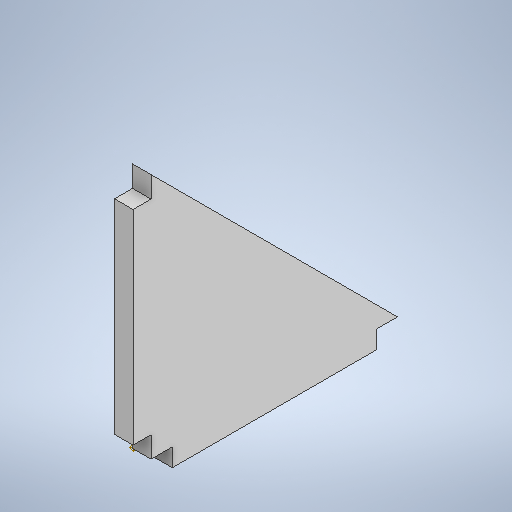
# Autodesk Inventor part: supporter
Saved by Autodesk Inventor 2025 (Build 290162000, 162)
## iProperties
Created: 2024-04-06
Part Number: supporter
Material: 일반
Document SubType Name: Modeling
Designer: gmsee
Density: 1 g/cm^3
Appearance: 기본값
Author: gmsee
Autodesk Inventor part; units mm, degrees
ref_plane "YZ Plane" through (0, 0, 0) normal (1, 0, 0) x (0, 1, 0)
ref_plane "XZ Plane" through (0, 0, 0) normal (0, 1, 0) x (-1, 0, 0)
ref_plane "XY Plane" through (0, 0, 0) normal (0, 0, 1) x (1, 0, 0)
sketch "스케치1" plane through (0, 0, 0) normal (1, 0, 0) x (0, 1, 0)
  line L0 (0, -46.5) -> (46.5, 0)
  line L1 (0, -4) -> (-3.4, -4)
  line L2 (-3.4, -4) -> (-3.4, -42.5)
  line L3 (-3.4, -42.5) -> (0, -42.5)
  line L4 (0, 0) -> (0, -4)
  line L5 (0, -42.5) -> (0, -46.5)
  line L6 (42.5, 0) -> (42.5, 3.4)
  line L7 (42.5, 3.4) -> (4, 3.4)
  line L8 (4, 3.4) -> (4, 0)
  line L9 (46.5, 0) -> (42.5, 0)
  line L10 (4, 0) -> (0, 0)
  point P0 (4, 1.7)
  point P1 (0, -44.5)
  dimension "d1" = 46.5
  dimension "d2" = 38.5
  dimension "d4" = 38.5
  dimension "d5" = 3.4
  dimension "d6" = 4
  dimension "d7" = 3.4
  dimension "d8" = 46.5
  constraints: 22 end point, 10 perpendicular, 3 horizontal, 2 midpoint, 1 coincident, 1 vertical
  measures "d1" distance of L4.start L0.start
  measures "d2" distance of L1.end L2.end
  measures "d4" distance of L6.end L7.end
  measures "d5" distance of L6.start L6.end
  measures "d6" distance from line of L4 point (4, 1.7)
  measures "d7" distance of L2.end L3.end
  measures "d8" horizontal distance of point (0, -44.5) L0.end
extrude "돌출1" add sketch "스케치1" along normal blind 3.5
